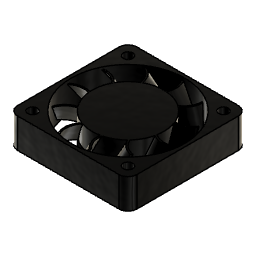
风扇 v1 (Autodesk Fusion 360 design; units mm, degrees)
Autodesk Fusion 360 part; units mm, degrees
sketch "草图1" plane through (0, 0, 0) normal (0, 0, 1) x (1, 0, 0)
  line L0 (3, 0) -> (37, 0)
  line L1 (40, 3) -> (40, 37)
  line L2 (37, 40) -> (3, 40)
  line L3 (0, 37) -> (0, 3)
  line L4 (46, 20) -> (-14, 20)
  line L5 (20, -15) -> (20, 49)
  circle A0 centre (36, 4) radius 1.6
  circle A1 centre (4, 4) radius 1.6
  circle A2 centre (36, 36) radius 1.6
  circle A3 centre (4, 36) radius 1.6
  arc A4 (37, 0) -> (40, 3) centre (37, 3) ccw
  arc A5 (0, 3) -> (3, 0) centre (3, 3) ccw
  arc A6 (3, 40) -> (0, 37) centre (3, 37) ccw
  arc A7 (40, 37) -> (37, 40) centre (37, 37) ccw
  point P0 (40, 0)
  point P1 (40, 40)
  dimension "d1" = 40
  dimension "d2" = 40
  dimension "d3" = 3.2
  dimension "d4" = 32
  dimension "d5" = 32
  dimension "d6" = 3
  constraint horizontal L0
  constraint vertical L1
  constraint horizontal L2
  constraint vertical L3
  constraint perpendicular L3 L4
  constraint vertical L5
  constraint symmetric L0 L2 L4
  constraint symmetric L5 A0 A1
  constraint symmetric L4 A0 A2
  constraint symmetric L4 A1 A3
  constraint coincident P0 L1
  constraint tangent L0 A4
  constraint tangent L1 A4
  constraint coincident origin L0
  constraint coincident origin L3
  constraint tangent L0 A5
  constraint tangent L3 A5
  constraint equal A4 A5
  constraint tangent L2 A6
  constraint tangent L3 A6
  constraint equal A4 A6
  constraint coincident P1 L1
  constraint coincident P1 L2
  constraint tangent L1 A7
  constraint tangent L2 A7
  constraint equal A4 A7
  measures "d1" distance of origin P0
  measures "d2" distance of P0 P1
  measures "d3" diameter of A0
  measures "d4" distance of A0.centre A1.centre
  measures "d5" distance of A0.centre A2.centre
  measures "d6" radius of A4
extrude "拉伸1" add sketch "草图1" along normal blind 10 makes body 1
sketch "草图2" plane through (0, 0, 10) normal (0, 0, 1) x (-1, 0, 0)
  circle A0 centre (-4, -4) radius 1.6
  circle A1 centre (-36, -36) radius 1.6
  circle A2 centre (-4, -36) radius 1.6
  circle A3 centre (-36, -4) radius 1.6
  arc A4 (-40, -37) -> (-37, -40) centre (-37, -37) ccw
  line L0 (-37, -40) -> (-3, -40)
  arc A5 (-3, -40) -> (0, -37) centre (-3, -37) ccw
  line L1 (0, -37) -> (0, -3)
  arc A6 (0, -3) -> (-3, 0) centre (-3, -3) ccw
  line L2 (-3, 0) -> (-37, 0)
  arc A7 (-37, 0) -> (-40, -3) centre (-37, -3) ccw
  line L3 (-40, -3) -> (-40, -37)
  circle A8 centre (-20, -20) radius 19
  dimension "d9" = 38
  dimension "d10" = 20
  dimension "d11" = 20
  measures "d9" diameter of A8
  measures "d10" distance of L1 A8.centre
  measures "d11" distance of L0 A8.centre
extrude "拉伸2" cut sketch "草图2" against normal blind 9 contours A8 bodies 1
sketch "草图3" plane through (0, 0, 1) normal (0, 0, 1) x (-1, 0, 0)
  circle A0 centre (-20, -20) radius 19
  circle A1 centre (-20, -20) radius 12
  circle A2 centre (-20, -20) radius 19
  line L0 (-8.1113, -18.3694) -> (-1.0701, -18.3694)
  line L1 (-1.0494, -21.3694) -> (-8.0784, -21.3694)
  line L2 (-27.3565, -10.5194) -> (-30.8771, -4.4215)
  line L3 (-28.2894, -2.9036) -> (-24.7749, -8.9909)
  line L4 (-24.5322, -31.1112) -> (-28.0528, -37.2091)
  line L5 (-30.6612, -35.727) -> (-27.1467, -29.6397)
  dimension "d14" = 24
  dimension "d15" = 38
  dimension "d17" = 3
  dimension "d19" = 360
  constraint concentric A0 A1
  constraint concentric A1 A2
  constraint horizontal L0
  constraint horizontal L1
  constraint coincident A0 L0.end
  constraint coincident A0 L1.start
  constraint coincident A1 L0.start
  constraint coincident A1 L1.end
  measures "d14" diameter of A1
  measures "d15" diameter of A2
  measures "d17" distance of L0 L1
extrude "拉伸3" cut sketch "草图3" against normal blind 1 contours A0 A1 A2 L0 L3 | A0 A1 A2 L1 L4 | A0 A1 A2 L2 L5 bodies 1
ref_plane "工作平面1" through (16.5028, 20.0563, 3) normal (0, 0, 1) x (-1, 0, 0)
sketch "草图4" plane through (16.5028, 20.0563, 3) normal (0, 0, 1) x (1, 0, 0)
  line L0 (14.3743, -15.6348) -> (10.8537, -9.537)
  arc A0 (10.8537, -9.537) -> (10.6439, 9.5834) centre (3.4972, -0.0563) ccw
  line L1 (10.6439, 9.5834) -> (14.1584, 15.6706)
  arc A1 (14.1584, 15.6706) -> (11.55, 17.1527) centre (3.4972, -0.0563) ccw
  line L2 (11.55, 17.1527) -> (8.0294, 11.0549)
  arc A2 (8.0294, 11.0549) -> (-8.4244, 1.3131) centre (3.4972, -0.0563) ccw
  line L3 (-8.4244, 1.3131) -> (-15.4534, 1.3131)
  arc A3 (-15.4534, 1.3131) -> (-15.4327, -1.6869) centre (3.4972, -0.0563) ccw
  line L4 (-15.4327, -1.6869) -> (-8.3915, -1.6869)
  arc A4 (-8.3915, -1.6869) -> (8.2721, -11.0655) centre (3.4972, -0.0563) ccw
  line L5 (8.2721, -11.0655) -> (11.7866, -17.1527)
  arc A5 (11.7866, -17.1527) -> (14.3743, -15.6348) centre (3.4972, -0.0563) ccw
  circle A6 centre (3.4972, -0.0563) radius 12
  dimension "d23" = 24
  constraint concentric A0 A6
  measures "d23" diameter of A6
extrude "拉伸4" add sketch "草图4" along normal blind 7 separate body contours A0 A2 A4 A6 makes body 2
sketch "草图5" plane through (16.5028, 20.0563, 3) normal (0, 0, 1) x (1, 0, 0)
  circle A0 centre (3.4972, -0.0563) radius 12
  arc A1 (2.9337, 11.9304) -> (1.7651, 17.8601) centre (-4.9485, 13.457) ccw
  arc A2 (3.4449, 11.9435) -> (2.3281, 17.9057) centre (-4.9485, 13.457) ccw
  line L0 (2.9337, 11.9304) -> (3.4449, 11.9435)
  arc A3 (2.3281, 17.9057) -> (1.7651, 17.8601) centre (3.4972, -0.0563) ccw
  dimension "d27" = 36
  constraint coincident A0 A1.start
  constraint concentric A0 A3
  constraint concentric A1 A2
  constraint coincident A0 A2.start
  measures "d27" diameter of A3
sketch "草图6" plane through (0, 0, 10) normal (0, 0, 1) x (-1, 0, 0)
  circle A0 centre (-20, -20) radius 12
  arc A1 (-15.9405, -31.2925) -> (-13.3932, -36.7436) centre (-9.8762, -31.7794) ccw
  arc A2 (-16.4525, -31.4636) -> (-13.9489, -36.9524) centre (-9.8762, -31.7794) ccw
  arc A3 (-13.9489, -36.9524) -> (-13.3932, -36.7436) centre (-20, -20) ccw
  line L0 (-15.9405, -31.2925) -> (-16.4525, -31.4636)
  dimension "d29" = 36
  constraint coincident A0 A1.start
  constraint concentric A0 A3
  constraint concentric A1 A2
  constraint coincident A0 A2.start
  measures "d29" diameter of A3
loft "放样1" add profiles "草图5", "草图6" section 1 contours A0 A1 A2 A3 section 2 contours A0 A1 A2 A3 separate body makes body 3
pattern_circular "C-阵列1" count 11 over 360 about axis through (20, 20, 10) along (0, 0, 1) of bodies 3 makes body 4 at (9.9921, 31.7509, 5.3333) makes body 5 at (5.2278, 24.4748, 5.3333) makes body 6 at (5.1536, 15.778, 5.3333) makes body 7 at (9.793, 8.4216, 5.3333) makes body 8 at (17.673, 4.7413, 5.3333) makes body 9 at (26.2919, 5.9055, 5.3333) makes body 10 at (32.9131, 11.5446, 5.3333) makes body 11 at (35.4345, 19.8683, 5.3333) makes body 12 at (33.0556, 28.2337, 5.3333) makes body 13 at (26.5316, 33.985, 5.3333)
combine "合并1" operation add target body 2 tool bodies 3 5 11 7 13 4 12 10 6 8 9
copy_body "实体->零部件1" bodies 1 removing the originals makes body 14 in component "Component'"
copy_body "实体->零部件2" bodies 2 removing the originals makes body 15 in component "Component''"
component "Component'" placed x (1, 0, 0) y (0, 1, 0) z (0, 0, 1) at (0, 0, 0)
component "Component''" placed x (1, 0, 0) y (0, 1, 0) z (0, 0, 1) at (0, 0, 0)
